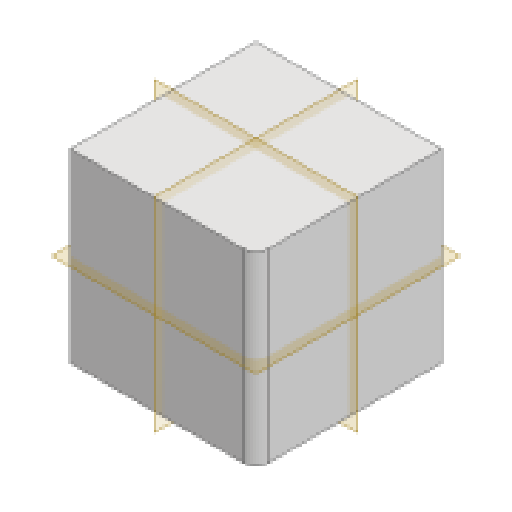
# Autodesk Inventor part: кубик
Saved by Autodesk Inventor 2023.2 (Build 272271030, 271C)
## iProperties
Created: 2025-04-24
Part Number: кубик
Material: Типовые
Document SubType Name: Modeling
Designer: Коноваленко
Density: 1 g/cm^3
Appearance: По умолчанию
Author: Коноваленко
Autodesk Inventor part; units mm, degrees
sketch "Эскиз1" plane through (0, 0, 0) normal (0, 1, 0) x (-1, 0, 0)
  line L0 (15, 15) -> (-15, 15)
  line L1 (-15, 15) -> (-15, -15)
  line L2 (-15, -15) -> (15, -15)
  line L3 (15, -15) -> (15, 15)
  line L4 (15, 15) -> (-15, -15) construction
  line L5 (-15, 15) -> (15, -15) construction
  point P0 (0, 0)
  dimension "d0" = 30
  dimension "d1" = 30
  constraints: 12 end point, 2 midpoint, 2 parallel, 1 horizontal, 1 perpendicular
  measures "d0" distance of L1.end L2.end
  measures "d1" distance of L0.end L1.end
extrude "Выдавливание1" add sketch "Эскиз1" along normal mid plane 30
sketch "Эскиз2" plane through (-15, -15, 15) normal (-1, 0, 0) x (0, 0, 1)
  arc A0 (0, 0) -> (-30, 30) centre (-30, 0) ccw projected
  line L0 (-30, 30) -> (0, 30) projected
  line L1 (0, 0) -> (0, 30) projected
  line L2 (-30, 30) -> (-30, 0) projected
  point P0 (-15, 15)
revolve "Вращение1" cut sketch "Эскиз2" angle 90 about axis through (-15, 15, -15) along (0, -1, 0)
